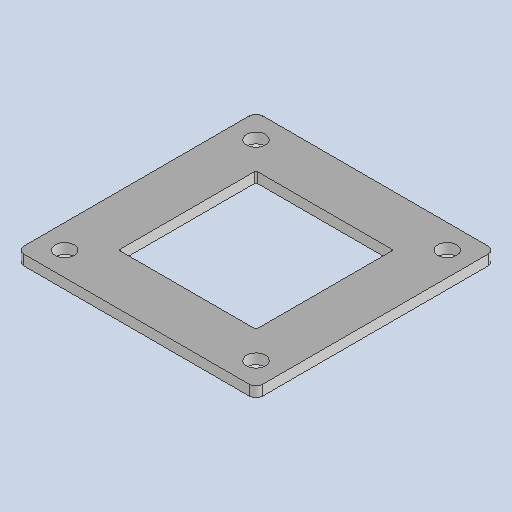
# Autodesk Inventor part: KND-1425 DrSysB Way FLANGE 01
Saved by Autodesk Inventor 2026.2 (Build 302298000, 298)
## iProperties
Created: 2025-06-24
Part Number: KND-1425 DrSysB Way FLANGE 01
Material: Stainless Steel
Document SubType Name: Sheet Metal
Designer: admin
Mass: 62.1684 g
Surface Area: 64.55 cm^2
Volume: 7.77105 cm^3
Density: 8 g/cm^3
Flat Pattern Width: 7 cm
Flat Pattern Length: 7 cm
Flat Pattern Area: 49 cm^2
Sheet Metal Rule: AISI304 2mm Die16
Sheet Metal Width: 70,000 mm
Sheet Metal Length: 70,000 mm
Sheet Metal Area: 4900,000 mm^2
Appearance: Default
Author: user
Autodesk Inventor part; units mm, degrees
ref_plane "YZ Plane" through (0, 0, 0) normal (1, 0, 0) x (0, 1, 0)
ref_plane "XZ Plane" through (0, 0, 0) normal (0, 1, 0) x (-1, 0, 0)
ref_plane "XY Plane" through (0, 0, 0) normal (0, 0, 1) x (1, 0, 0)
sketch "Sketch1" plane through (0, 0, 0) normal (0, 0, 1) x (1, 0, 0)
  line L0 (-35, -35) -> (35, -35)
  line L1 (35, -35) -> (35, 35)
  line L2 (35, 35) -> (-35, 35)
  line L3 (-35, 35) -> (-35, -35)
  line L4 (-35, -35) -> (35, 35) construction
  line L5 (35, -35) -> (-35, 35) construction
  line L6 (20.1, -20.1) -> (-20.1, -20.1)
  line L7 (-20.1, -20.1) -> (-20.1, 20.1)
  line L8 (-20.1, 20.1) -> (20.1, 20.1)
  line L9 (20.1, 20.1) -> (20.1, -20.1)
  line L10 (20.1, -20.1) -> (-20.1, 20.1) construction
  line L11 (-20.1, -20.1) -> (20.1, 20.1) construction
  circle A0 centre (-28, -28) radius 2.75
  circle A1 centre (28, -28) radius 2.75
  circle A2 centre (28, 28) radius 2.75
  circle A3 centre (-28, 28) radius 2.75
  line L12 (30.75, 30.75) -> (-30.75, 30.75) construction
  line L13 (-30.75, 30.75) -> (-30.75, -30.75) construction
  line L14 (-30.75, -30.75) -> (30.75, -30.75) construction
  line L15 (30.75, -30.75) -> (30.75, 30.75) construction
  line L16 (30.75, 30.75) -> (-30.75, -30.75) construction
  line L17 (-30.75, 30.75) -> (30.75, -30.75) construction
  line L18 (28, 28) -> (-28, 28) construction
  line L19 (-28, 28) -> (-28, -28) construction
  line L20 (-28, -28) -> (28, -28) construction
  line L21 (28, -28) -> (28, 28) construction
  line L22 (28, 28) -> (-28, -28) construction
  line L23 (-28, 28) -> (28, -28) construction
  point P0 (0, 0)
  dimension "d172" = 40.2
  dimension "d190" = 5.5
  dimension "d191" = 56
  dimension "d192" = 70
  measures "d172" distance of L7.end L8.end
  measures "d190" diameter of A0
  measures "d191" distance of L19.end L20.end
  measures "d192" distance of L2.end L0.start
extrude "Plate5" add sketch "Sketch1" along normal blind 3
fillet "Corner Round1" radius 2 4 edges at (35, 35, 1.5) (-35, 35, 1.5) (-35, -35, 1.5) (35, -35, 1.5)
fillet "Corner Round2" radius 0.5 4 edges at (-20.1, 20.1, 1.5) (-20.1, -20.1, 1.5) (20.1, -20.1, 1.5) (20.1, 20.1, 1.5)
derived "KND-1401 DrSysB DIMentions 01.ipt"
body "Solid3"
